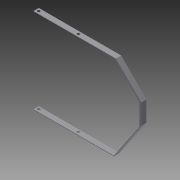
# Autodesk Inventor part: 4barRoundedBar
Saved by Autodesk Inventor 2015 SP1 (Build 190203100, 203)
## iProperties
Created: 2015-02-16
Part Number: 4barRoundedBar
Material: Generic
Document SubType Name: Modeling
Designer: 55221
Density: 1 g/cm^3
Appearance: Default
Author: 55221
Autodesk Inventor part; units mm, degrees
ref_plane "YZ Plane" through (0, 0, 0) normal (1, 0, 0) x (0, 1, 0)
ref_plane "XZ Plane" through (0, 0, 0) normal (0, 1, 0) x (-1, 0, 0)
ref_plane "XY Plane" through (0, 0, 0) normal (0, 0, 1) x (1, 0, 0)
sketch "Sketch9" plane through (0, 0, 0) normal (0, 0, 1) x (1, 0, 0)
  line L0 (0, 0) -> (395.8194, 0)
  line L1 (387.9689, -2.54) -> (508, -123.4756)
  line L2 (508, -123.4756) -> (508, -228.3729)
  line L3 (517.1565, -218.6006) -> (386.5644, -411.48)
  line L4 (386.5644, -411.48) -> (0, -411.48)
  line L5 (0, -411.48) -> (0, -408.94)
  line L6 (0, -408.94) -> (385.7441, -408.94)
  line L7 (385.7441, -408.94) -> (508, -228.3729)
  line L8 (517.1565, -218.6006) -> (517.1565, -122.2514)
  line L9 (517.1565, -122.2514) -> (395.8194, 0)
  line L10 (387.9689, -2.54) -> (0, -2.54)
  line L11 (0, -2.54) -> (0, 0)
  dimension "d32" = 508
  dimension "d35" = 406.4
  dimension "d36" = 2.54
  dimension "d37" = 2.54
  constraints: 24 end point, 5 parallel, 4 perpendicular, 1 horizontal, 1 point on line
  measures "d32" distance between parallel lines of L11 L2
  measures "d35" distance between parallel lines of L6 L10
  measures "d36" distance between parallel lines of L4 L6
  measures "d37" distance between parallel lines of L10 L0
extrude "Extrusion6" add sketch "Sketch9" along normal blind 25.4
hole "Hole1" at (12.7, 0, 12.7) direction (0, -1, 0) diameter 12.7 end through all
hole "Hole2" at (203.2, 0, 12.7) direction (0, -1, 0) diameter 12.7 end through all
body "Solid2"
